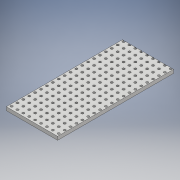
# Autodesk Inventor part: Lochrasterplatine
Saved by Autodesk Inventor 2017.3 (Build 213257000, 257)
## iProperties
Part Number: Lochrasterplatine
Material: Generisch
Document SubType Name: Modeling
Designer: Enno
Density: 1 g/cm^3
Appearance: Vorgabe
Author: Enno
Autodesk Inventor part; units mm, degrees
ref_plane "YZ Plane" through (0, 0, 0) normal (1, 0, 0) x (0, 1, 0)
ref_plane "XZ Plane" through (0, 0, 0) normal (0, 1, 0) x (-1, 0, 0)
ref_plane "XY Plane" through (0, 0, 0) normal (0, 0, 1) x (1, 0, 0)
sketch "Skizze1" plane through (0, 0, 0) normal (0, 0, 1) x (1, 0, 0)
  line L0 (0, 0) -> (30, 0)
  line L1 (30, 0) -> (30, 50)
  line L2 (30, 50) -> (0, 50)
  line L3 (0, 50) -> (0, 0)
  dimension "d0" = 30
  dimension "d1" = 50
  constraints: 8 end point, 2 parallel, 1 horizontal, 1 perpendicular
  measures "d0" distance of L2.end L1.end
  measures "d1" distance of L1.end L0.end
extrude "Extrusion1" add sketch "Skizze1" against normal blind 1.5
sketch "Skizze2" plane through (0, 0, 0) normal (0, 0, 1) x (1, 0, 0)
  line L0 (30, 0) -> (0, 0) projected
  line L1 (0, 0) -> (37.7707, 0) construction
  line L2 (0, 0) -> (0, 66.1095) construction
  point P0 (1.27, 1.27)
  point P1 (3.81, 1.27)
  point P2 (6.35, 1.27)
  point P3 (8.89, 1.27)
  point P4 (11.43, 1.27)
  point P5 (13.97, 1.27)
  point P6 (16.51, 1.27)
  point P7 (19.05, 1.27)
  point P8 (21.59, 1.27)
  point P9 (24.13, 1.27)
  point P10 (26.67, 1.27)
  point P11 (29.21, 1.27)
  point P12 (1.27, 3.81)
  point P13 (3.81, 3.81)
  point P14 (6.35, 3.81)
  point P15 (8.89, 3.81)
  point P16 (11.43, 3.81)
  point P17 (13.97, 3.81)
  point P18 (16.51, 3.81)
  point P19 (19.05, 3.81)
  point P20 (21.59, 3.81)
  point P21 (24.13, 3.81)
  point P22 (26.67, 3.81)
  point P23 (29.21, 3.81)
  point P24 (1.27, 6.35)
  point P25 (3.81, 6.35)
  point P26 (6.35, 6.35)
  point P27 (8.89, 6.35)
  point P28 (11.43, 6.35)
  point P29 (13.97, 6.35)
  point P30 (16.51, 6.35)
  point P31 (19.05, 6.35)
  point P32 (21.59, 6.35)
  point P33 (24.13, 6.35)
  point P34 (26.67, 6.35)
  point P35 (29.21, 6.35)
  point P36 (1.27, 8.89)
  point P37 (3.81, 8.89)
  point P38 (6.35, 8.89)
  point P39 (8.89, 8.89)
  point P40 (11.43, 8.89)
  point P41 (13.97, 8.89)
  point P42 (16.51, 8.89)
  point P43 (19.05, 8.89)
  point P44 (21.59, 8.89)
  point P45 (24.13, 8.89)
  point P46 (26.67, 8.89)
  point P47 (29.21, 8.89)
  point P48 (1.27, 11.43)
  point P49 (3.81, 11.43)
  point P50 (6.35, 11.43)
  point P51 (8.89, 11.43)
  point P52 (11.43, 11.43)
  point P53 (13.97, 11.43)
  point P54 (16.51, 11.43)
  point P55 (19.05, 11.43)
  point P56 (21.59, 11.43)
  point P57 (24.13, 11.43)
  point P58 (26.67, 11.43)
  point P59 (29.21, 11.43)
  point P60 (1.27, 13.97)
  point P61 (3.81, 13.97)
  point P62 (6.35, 13.97)
  point P63 (8.89, 13.97)
  point P64 (11.43, 13.97)
  point P65 (13.97, 13.97)
  point P66 (16.51, 13.97)
  point P67 (19.05, 13.97)
  point P68 (21.59, 13.97)
  point P69 (24.13, 13.97)
  point P70 (26.67, 13.97)
  point P71 (29.21, 13.97)
  point P72 (1.27, 16.51)
  point P73 (3.81, 16.51)
  point P74 (6.35, 16.51)
  point P75 (8.89, 16.51)
  point P76 (11.43, 16.51)
  point P77 (13.97, 16.51)
  point P78 (16.51, 16.51)
  point P79 (19.05, 16.51)
  point P80 (21.59, 16.51)
  point P81 (24.13, 16.51)
  point P82 (26.67, 16.51)
  point P83 (29.21, 16.51)
  point P84 (1.27, 19.05)
  point P85 (3.81, 19.05)
  point P86 (6.35, 19.05)
  point P87 (8.89, 19.05)
  point P88 (11.43, 19.05)
  point P89 (13.97, 19.05)
  point P90 (16.51, 19.05)
  point P91 (19.05, 19.05)
  point P92 (21.59, 19.05)
  point P93 (24.13, 19.05)
  point P94 (26.67, 19.05)
  point P95 (29.21, 19.05)
  point P96 (1.27, 21.59)
  point P97 (3.81, 21.59)
  point P98 (6.35, 21.59)
  point P99 (8.89, 21.59)
  point P100 (11.43, 21.59)
  point P101 (13.97, 21.59)
  point P102 (16.51, 21.59)
  point P103 (19.05, 21.59)
  point P104 (21.59, 21.59)
  point P105 (24.13, 21.59)
  point P106 (26.67, 21.59)
  point P107 (29.21, 21.59)
  point P108 (1.27, 24.13)
  point P109 (3.81, 24.13)
  point P110 (6.35, 24.13)
  point P111 (8.89, 24.13)
  point P112 (11.43, 24.13)
  point P113 (13.97, 24.13)
  point P114 (16.51, 24.13)
  point P115 (19.05, 24.13)
  point P116 (21.59, 24.13)
  point P117 (24.13, 24.13)
  point P118 (26.67, 24.13)
  point P119 (29.21, 24.13)
  point P120 (1.27, 26.67)
  point P121 (3.81, 26.67)
  point P122 (6.35, 26.67)
  point P123 (8.89, 26.67)
  point P124 (11.43, 26.67)
  point P125 (13.97, 26.67)
  point P126 (16.51, 26.67)
  point P127 (19.05, 26.67)
  point P128 (21.59, 26.67)
  point P129 (24.13, 26.67)
  point P130 (26.67, 26.67)
  point P131 (29.21, 26.67)
  point P132 (1.27, 29.21)
  point P133 (3.81, 29.21)
  point P134 (6.35, 29.21)
  point P135 (8.89, 29.21)
  point P136 (11.43, 29.21)
  point P137 (13.97, 29.21)
  point P138 (16.51, 29.21)
  point P139 (19.05, 29.21)
  point P140 (21.59, 29.21)
  point P141 (24.13, 29.21)
  point P142 (26.67, 29.21)
  point P143 (29.21, 29.21)
  point P144 (1.27, 31.75)
  point P145 (3.81, 31.75)
  point P146 (6.35, 31.75)
  point P147 (8.89, 31.75)
  point P148 (11.43, 31.75)
  point P149 (13.97, 31.75)
  point P150 (16.51, 31.75)
  point P151 (19.05, 31.75)
  point P152 (21.59, 31.75)
  point P153 (24.13, 31.75)
  point P154 (26.67, 31.75)
  point P155 (29.21, 31.75)
  point P156 (1.27, 34.29)
  point P157 (3.81, 34.29)
  point P158 (6.35, 34.29)
  point P159 (8.89, 34.29)
  point P160 (11.43, 34.29)
  point P161 (13.97, 34.29)
  point P162 (16.51, 34.29)
  point P163 (19.05, 34.29)
  point P164 (21.59, 34.29)
  point P165 (24.13, 34.29)
  point P166 (26.67, 34.29)
  point P167 (29.21, 34.29)
  point P168 (1.27, 36.83)
  point P169 (3.81, 36.83)
  point P170 (6.35, 36.83)
  point P171 (8.89, 36.83)
  point P172 (11.43, 36.83)
  point P173 (13.97, 36.83)
  point P174 (16.51, 36.83)
  point P175 (19.05, 36.83)
  point P176 (21.59, 36.83)
  point P177 (24.13, 36.83)
  point P178 (26.67, 36.83)
  point P179 (29.21, 36.83)
  point P180 (1.27, 39.37)
  point P181 (3.81, 39.37)
  point P182 (6.35, 39.37)
  point P183 (8.89, 39.37)
  point P184 (11.43, 39.37)
  point P185 (13.97, 39.37)
  point P186 (16.51, 39.37)
  point P187 (19.05, 39.37)
  point P188 (21.59, 39.37)
  point P189 (24.13, 39.37)
  point P190 (26.67, 39.37)
  point P191 (29.21, 39.37)
  point P192 (1.27, 41.91)
  point P193 (3.81, 41.91)
  point P194 (6.35, 41.91)
  point P195 (8.89, 41.91)
  point P196 (11.43, 41.91)
  point P197 (13.97, 41.91)
  point P198 (16.51, 41.91)
  point P199 (19.05, 41.91)
  dimension "d4" = 1.27
  dimension "d5" = 1.27
  dimension "d8" = 2.54
  dimension "d11" = 2.54
  constraints: 4 end point, 2 horizontal, 1 perpendicular, 1 vertical, 239 other
  measures "d4" distance from line of L2 point (1.27, 1.27)
  measures "d5" distance from line of L0 point (1.27, 1.27)
  measures "d8" distance of point (1.27, 1.27) point (3.81, 1.27)
  measures "d11" distance of point (1.27, 1.27) point (1.27, 3.81)
hole "Bohrung1" at (1.27, 1.27, 0) at (3.81, 1.27, 0) at (6.35, 1.27, 0) at (8.89, 1.27, 0) at (11.43, 1.27, 0) at (13.97, 1.27, 0) at (16.51, 1.27, 0) at (19.05, 1.27, 0) at (21.59, 1.27, 0) at (24.13, 1.27, 0) at (26.67, 1.27, 0) at (29.21, 1.27, 0) at (1.27, 3.81, 0) at (3.81, 3.81, 0) at (6.35, 3.81, 0) at (8.89, 3.81, 0) at (11.43, 3.81, 0) at (13.97, 3.81, 0) at (16.51, 3.81, 0) at (19.05, 3.81, 0) at (21.59, 3.81, 0) at (24.13, 3.81, 0) at (26.67, 3.81, 0) at (29.21, 3.81, 0) at (1.27, 6.35, 0) at (3.81, 6.35, 0) at (6.35, 6.35, 0) at (8.89, 6.35, 0) at (11.43, 6.35, 0) at (13.97, 6.35, 0) at (16.51, 6.35, 0) at (19.05, 6.35, 0) at (21.59, 6.35, 0) at (24.13, 6.35, 0) at (26.67, 6.35, 0) at (29.21, 6.35, 0) at (1.27, 8.89, 0) at (3.81, 8.89, 0) at (6.35, 8.89, 0) at (8.89, 8.89, 0) at (11.43, 8.89, 0) at (13.97, 8.89, 0) at (16.51, 8.89, 0) at (19.05, 8.89, 0) at (21.59, 8.89, 0) at (24.13, 8.89, 0) at (26.67, 8.89, 0) at (29.21, 8.89, 0) at (1.27, 11.43, 0) at (3.81, 11.43, 0) direction (0, 0, -1) diameter 1 end through all and at (6.35, 11.43, 0) (8.89, 11.43, 0) (11.43, 11.43, 0) (13.97, 11.43, 0) (16.51, 11.43, 0) (19.05, 11.43, 0) (21.59, 11.43, 0) (24.13, 11.43, 0) (26.67, 11.43, 0) (29.21, 11.43, 0) (1.27, 13.97, 0) (3.81, 13.97, 0) (6.35, 13.97, 0) (8.89, 13.97, 0) (11.43, 13.97, 0) (13.97, 13.97, 0) (16.51, 13.97, 0) (19.05, 13.97, 0) (21.59, 13.97, 0) (24.13, 13.97, 0) (26.67, 13.97, 0) (29.21, 13.97, 0) (1.27, 16.51, 0) (3.81, 16.51, 0) (6.35, 16.51, 0) (8.89, 16.51, 0) (11.43, 16.51, 0) (13.97, 16.51, 0) (16.51, 16.51, 0) (19.05, 16.51, 0) (21.59, 16.51, 0) (24.13, 16.51, 0) (26.67, 16.51, 0) (29.21, 16.51, 0) (1.27, 19.05, 0) (3.81, 19.05, 0) (6.35, 19.05, 0) (8.89, 19.05, 0) (11.43, 19.05, 0) (13.97, 19.05, 0) (16.51, 19.05, 0) (19.05, 19.05, 0) (21.59, 19.05, 0) (24.13, 19.05, 0) (26.67, 19.05, 0) (29.21, 19.05, 0) (1.27, 21.59, 0) (3.81, 21.59, 0) (6.35, 21.59, 0) (8.89, 21.59, 0) (11.43, 21.59, 0) (13.97, 21.59, 0) (16.51, 21.59, 0) (19.05, 21.59, 0) (21.59, 21.59, 0) (24.13, 21.59, 0) (26.67, 21.59, 0) (29.21, 21.59, 0) (1.27, 24.13, 0) (3.81, 24.13, 0) (6.35, 24.13, 0) (8.89, 24.13, 0) (11.43, 24.13, 0) (13.97, 24.13, 0) (16.51, 24.13, 0) (19.05, 24.13, 0) (21.59, 24.13, 0) (24.13, 24.13, 0) (26.67, 24.13, 0) (29.21, 24.13, 0) (1.27, 26.67, 0) (3.81, 26.67, 0) (6.35, 26.67, 0) (8.89, 26.67, 0) (11.43, 26.67, 0) (13.97, 26.67, 0) (16.51, 26.67, 0) (19.05, 26.67, 0) (21.59, 26.67, 0) (24.13, 26.67, 0) (26.67, 26.67, 0) (29.21, 26.67, 0) (1.27, 29.21, 0) (3.81, 29.21, 0) (6.35, 29.21, 0) (8.89, 29.21, 0) (11.43, 29.21, 0) (13.97, 29.21, 0) (16.51, 29.21, 0) (19.05, 29.21, 0) (21.59, 29.21, 0) (24.13, 29.21, 0) (26.67, 29.21, 0) (29.21, 29.21, 0) (1.27, 31.75, 0) (3.81, 31.75, 0) (6.35, 31.75, 0) (8.89, 31.75, 0) (11.43, 31.75, 0) (13.97, 31.75, 0) (16.51, 31.75, 0) (19.05, 31.75, 0) (21.59, 31.75, 0) (24.13, 31.75, 0) (26.67, 31.75, 0) (29.21, 31.75, 0) (1.27, 34.29, 0) (3.81, 34.29, 0) (6.35, 34.29, 0) (8.89, 34.29, 0) (11.43, 34.29, 0) (13.97, 34.29, 0) (16.51, 34.29, 0) (19.05, 34.29, 0) (21.59, 34.29, 0) (24.13, 34.29, 0) (26.67, 34.29, 0) (29.21, 34.29, 0) (1.27, 36.83, 0) (3.81, 36.83, 0) (6.35, 36.83, 0) (8.89, 36.83, 0) (11.43, 36.83, 0) (13.97, 36.83, 0) (16.51, 36.83, 0) (19.05, 36.83, 0) (21.59, 36.83, 0) (24.13, 36.83, 0) (26.67, 36.83, 0) (29.21, 36.83, 0) (1.27, 39.37, 0) (3.81, 39.37, 0) (6.35, 39.37, 0) (8.89, 39.37, 0) (11.43, 39.37, 0) (13.97, 39.37, 0) (16.51, 39.37, 0) (19.05, 39.37, 0) (21.59, 39.37, 0) (24.13, 39.37, 0) (26.67, 39.37, 0) (29.21, 39.37, 0) (1.27, 41.91, 0) (3.81, 41.91, 0) (6.35, 41.91, 0) (8.89, 41.91, 0) (11.43, 41.91, 0) (13.97, 41.91, 0) (16.51, 41.91, 0) (19.05, 41.91, 0) (21.59, 41.91, 0) (24.13, 41.91, 0) (26.67, 41.91, 0) (29.21, 41.91, 0) (1.27, 44.45, 0) (3.81, 44.45, 0) (6.35, 44.45, 0) (8.89, 44.45, 0) (11.43, 44.45, 0) (13.97, 44.45, 0) (16.51, 44.45, 0) (19.05, 44.45, 0) (21.59, 44.45, 0) (24.13, 44.45, 0) (26.67, 44.45, 0) (29.21, 44.45, 0) (1.27, 46.99, 0) (3.81, 46.99, 0) (6.35, 46.99, 0) (8.89, 46.99, 0) (11.43, 46.99, 0) (13.97, 46.99, 0) (16.51, 46.99, 0) (19.05, 46.99, 0) (21.59, 46.99, 0) (24.13, 46.99, 0) (26.67, 46.99, 0) (29.21, 46.99, 0) (1.27, 49.53, 0) (3.81, 49.53, 0) (6.35, 49.53, 0) (8.89, 49.53, 0) (11.43, 49.53, 0) (13.97, 49.53, 0) (16.51, 49.53, 0) (19.05, 49.53, 0) (21.59, 49.53, 0) (24.13, 49.53, 0) (26.67, 49.53, 0) (29.21, 49.53, 0)
sketch "Skizze3" plane through (0, 0, 0) normal (-1, 0, 0) x (0, 0, 1)
  line L0 (-1.5, 49.03) -> (-1.5, 50) projected
  line L1 (0, 0) -> (-1.5, 0)
  line L2 (-1.5, 0) -> (-1.5, 50)
  line L3 (-1.5, 50) -> (0, 50)
  line L4 (0, 50) -> (0, 0)
  constraints: 8 end point, 2 parallel, 1 horizontal, 1 perpendicular
extrude "Extrusion2" cut sketch "Skizze3" against normal blind 7.9
